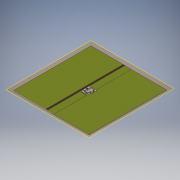
# Autodesk Inventor part: Umgebung
Saved by Autodesk Inventor 2019 (Build 230136000, 136)
## iProperties
Created: 2019-05-04
Part Number: Umgebung
Material: Generisch
Document SubType Name: Modeling
Designer: niede
Density: 1 g/cm^3
Appearance: Default
Author: niede
Autodesk Inventor part; units mm, degrees
ref_plane "YZ Plane" through (0, 0, 0) normal (1, 0, 0) x (0, 1, 0)
ref_plane "XZ Plane" through (0, 0, 0) normal (0, 1, 0) x (-1, 0, 0)
ref_plane "XY Plane" through (0, 0, 0) normal (0, 0, 1) x (1, 0, 0)
sketch "Skizze2" plane through (0, 0, 0) normal (0, 1, 0) x (-1, 0, 0)
  line L0 (0, 0) -> (11230, 0)
  line L1 (11230, 0) -> (11230, -6920)
  line L2 (11230, -6920) -> (10230, -6920)
  line L3 (10230, -6920) -> (10230, -17740)
  line L4 (10230, -17740) -> (11230, -17740)
  line L5 (11230, -17740) -> (11230, -17980)
  line L6 (11230, -17980) -> (2740, -17980)
  line L7 (2740, -17980) -> (2740, -14980)
  line L8 (2740, -14980) -> (-1250, -14980)
  line L9 (-1250, -14980) -> (-1250, -8870)
  line L10 (-1250, -8870) -> (1180, -8870)
  line L11 (1180, -8870) -> (1180, -4980)
  line L12 (1180, -4980) -> (0, -4980)
  line L13 (0, -4980) -> (0, 0)
  line L14 (111230, 100000) -> (-101250, 100000)
  line L15 (-101250, 100000) -> (-101250, -117980)
  line L16 (-101250, -117980) -> (111230, -117980)
  line L17 (111230, -117980) -> (111230, 100000)
  dimension "d0" = 11230
  dimension "d1" = 6920
  dimension "d2" = 1000
  dimension "d3" = 10820
  dimension "d4" = 240
  dimension "d5" = 8490
  dimension "d6" = 3000
  dimension "d7" = 3990
  dimension "d8" = 6110
  dimension "d9" = 2430
  dimension "d10" = 3890
  dimension "d11" = 1180
  dimension "d12" = 11230
  dimension "d13" = 6920
  dimension "d14" = 100000
  dimension "d15" = 100000
  dimension "d16" = 100000
  dimension "d17" = 100000
  constraints: 36 end point, 10 perpendicular, 2 horizontal, 2 parallel, 2 point on line, 2 vertical
  measures "d0" distance of L0.start L0.end
  measures "d1" distance of L0.end L1.end
  measures "d2" distance of L1.end L2.end
  measures "d3" distance of L2.end L3.end
  measures "d4" distance of L4.end L5.end
  measures "d5" distance of L5.end L6.end
  measures "d6" distance of L6.end L7.end
  measures "d7" distance of L7.end L8.end
  measures "d8" distance of L8.end L9.end
  measures "d9" distance of L9.end L10.end
  measures "d10" distance of L10.end L11.end
  measures "d11" distance of L11.end L12.end
  measures "d12" distance from line of point (0, 0) L1
  measures "d13" distance from line of point (0, 0) L2
  measures "d14" distance between parallel lines of L17 L1
  measures "d15" distance between parallel lines of L15 L9
  measures "d16" distance between parallel lines of L6 L16
  measures "d17" distance between parallel lines of L0 L14
extrude "Haus_Senkung" add sketch "Skizze2" along normal blind 1700
sketch "Skizze3" plane through (0, 1700, 0) normal (0, 1, 0) x (1, 0, 0)
  line L0 (1250, 8870) -> (-1180, 8870) projected
  line L1 (-1180, 8870) -> (-1180, 4980) projected
  line L2 (0, 4980) -> (-1180, 4980) projected
  line L3 (4500, 4980) -> (4500, 8870)
  line L4 (4500, 8870) -> (1250, 8870)
  line L5 (3000, 4980) -> (3000, 2880)
  line L6 (3000, 2880) -> (1800, 2880)
  line L7 (1800, 2880) -> (1800, 4980)
  line L8 (0, 4980) -> (1800, 4980)
  line L9 (3000, 4980) -> (4500, 4980)
  dimension "d20" = 4500
  dimension "d47" = 1500
  dimension "d48" = 1200
  dimension "d49" = 2100
  constraints: 14 end point, 8 perpendicular, 2 horizontal, 1 collinear
  measures "d20" distance of L2.start L3.start
  measures "d47" distance between parallel lines of L5 L3
  measures "d48" distance between parallel lines of L5 L7
  measures "d49" distance of L6.end L7.end
extrude "Terrasse_Senkung_1" cut sketch "Skizze3" against normal blind 1400
sketch "Skizze4" plane through (1250, 0, -14980) normal (-1, 0, 0) x (0, 0, 1)
  line L0 (6110, 300) -> (6110, 1700) projected
  line L1 (0, 1700) -> (6110, 1700) projected
  line L2 (0, 0) -> (0, 1700) projected
  line L3 (6110, 500) -> (5760, 500)
  line L4 (5760, 500) -> (5760, 700)
  line L5 (5760, 700) -> (5410, 700)
  line L6 (5410, 700) -> (5410, 900)
  line L7 (5410, 900) -> (5060, 900)
  line L8 (5060, 900) -> (5060, 1100)
  line L9 (5060, 1100) -> (4710, 1100)
  line L10 (4710, 1100) -> (4710, 1300)
  line L11 (4710, 1300) -> (700, 1300)
  line L12 (700, 1300) -> (700, 1500)
  line L13 (700, 1500) -> (350, 1500)
  line L14 (350, 1500) -> (350, 1700)
  point P0 (14980, 0)
  dimension "d23" = 200
  dimension "d24" = 200
  dimension "d25" = 350
  dimension "d29" = 350
  constraints: 24 end point, 10 perpendicular, 8 parallel, 2 point on line, 1 horizontal, 1 vertical
  measures "d23" distance of L5.end L6.end
  measures "d24" distance from line of L3 L0.start
  measures "d25" distance of L4.end L5.end
  measures "d29" distance between parallel lines of L2 L14
extrude "Terrasse_Treppe_Rechts" cut sketch "Skizze4" against normal blind 1200
sketch "Skizze8" plane through (0, 1700, 0) normal (0, 1, 0) x (1, 0, 0)
  line L0 (2450, 14630) -> (2450, 8870) projected
  line L1 (2450, 8870) -> (4500, 8870) projected
  line L2 (4500, 8870) -> (4500, 4980) projected
  line L3 (4500, 4980) -> (3000, 4980) projected
  line L4 (3000, 4980) -> (3000, 2880) projected
  line L5 (2450, 9870) -> (5500, 9870)
  line L6 (5500, 9870) -> (5500, 3980)
  line L7 (5500, 3980) -> (3300, 3980)
  line L8 (3300, 3980) -> (3300, 4980)
  dimension "d50" = 1000
  dimension "d51" = 1000
  dimension "d52" = 1000
  dimension "d53" = 300
  constraints: 8 end point, 3 perpendicular, 2 point on line, 1 horizontal
  measures "d50" distance between parallel lines of L1 L5
  measures "d51" distance between parallel lines of L2 L6
  measures "d52" distance between parallel lines of L3 L7
  measures "d53" distance between parallel lines of L4 L8
extrude "Terrasse_Senkung_2" cut sketch "Skizze8" against normal blind 700
sketch "Skizze5" plane through (-2740, 0, -14980) normal (0, 0, 1) x (1, 0, 0)
  line L0 (3990, 0) -> (0, 0) projected
  line L1 (0, 1700) -> (3990, 1700) projected
  line L2 (0, 0) -> (0, 1700) projected
  line L3 (1350, 500) -> (1350, 700)
  line L4 (1350, 700) -> (1700, 700)
  line L5 (1700, 700) -> (1700, 900)
  line L6 (1700, 900) -> (2050, 900)
  line L7 (2050, 900) -> (2050, 1100)
  line L8 (2050, 1100) -> (2400, 1100)
  line L9 (2400, 1100) -> (2400, 1300)
  line L10 (2400, 1300) -> (2750, 1300)
  line L11 (2750, 1300) -> (2750, 1500)
  line L12 (2750, 1500) -> (3100, 1500)
  line L13 (3100, 1500) -> (3100, 1700)
  line L14 (1350, 500) -> (1000, 500)
  line L15 (1000, 500) -> (1000, 300)
  line L16 (1000, 300) -> (0, 300)
  point P0 (2740, 0)
  dimension "d32" = 200
  dimension "d33" = 1000
  dimension "d34" = 300
  dimension "d35" = 350
  constraints: 28 end point, 12 perpendicular, 11 parallel, 2 point on line, 1 horizontal
  measures "d32" distance of L3.start L3.end
  measures "d33" distance of L15.end L16.end
  measures "d34" distance between parallel lines of L0 L16
  measures "d35" distance of L3.start L14.end
extrude "Plattform_Treppe" cut sketch "Skizze5" against normal blind 1000
sketch "Skizze9" plane through (3000, 1700, -4980) normal (-1, 0, 0) x (0, 0, 1)
  line L0 (0, 0) -> (2100, 0) projected
  line L1 (0, 0) -> (0, -1400) projected
  line L2 (0, -1400) -> (2100, -1400) projected
  line L3 (2100, 0) -> (2100, -1400) projected
  line L4 (0, -1200) -> (300, -1200)
  line L5 (300, -1200) -> (300, -1000)
  line L6 (300, -1000) -> (600, -1000)
  line L7 (600, -1000) -> (600, -800)
  line L8 (600, -800) -> (900, -800)
  line L9 (900, -800) -> (900, -600)
  line L10 (900, -600) -> (1200, -600)
  line L11 (1200, -600) -> (1200, -400)
  line L12 (1200, -400) -> (1500, -400)
  line L13 (1500, -400) -> (1500, -200)
  line L14 (1500, -200) -> (1800, -200)
  line L15 (1800, -200) -> (1800, 0)
  point P0 (4980, -1700)
  dimension "d56" = 200
  dimension "d57" = 300
  constraints: 24 end point, 11 perpendicular, 10 parallel, 2 point on line, 1 horizontal
  measures "d56" distance of L14.end L15.end
  measures "d57" distance of L4.start L4.end
extrude "Terrasse_Treppe_Links" add sketch "Skizze9" along normal blind 1200 contours L0 L3 L2 L1 L4 L5 L6 L7 L8 L9 L10 L11 L12 L13 L14 L15
sketch "Skizze14" plane through (0, 1700, 0) normal (0, 1, 0) x (1, 0, 0)
  line L0 (-2740, 17980) -> (-2740, 15980) projected
  line L1 (-2740, 15980) -> (360, 15980) projected
  line L2 (360, 15980) -> (360, 14980) projected
  line L3 (360, 14980) -> (1250, 14980) projected
  line L4 (1250, 14980) -> (1250, 14630) projected
  line L5 (1250, 14630) -> (2450, 14630) projected
  line L6 (2450, 14630) -> (2450, 9870) projected
  line L7 (-2740, 17980) -> (6260, 17980)
  line L8 (6260, 17980) -> (6260, 13580)
  line L9 (6260, 13580) -> (2450, 13580)
  line L10 (2450, 10270) -> (2450, 14280) projected
  point P0 (0, 0)
  dimension "d79" = 9000
  dimension "d80" = 4400
  constraints: 6 end point, 2 perpendicular, 1 horizontal, 1 point on line
  measures "d79" distance of L0.start L7.end
  measures "d80" distance of L7.end L8.end
extrude "Plattform_Erhebung" add sketch "Skizze14" along normal blind 200
sketch "Skizze10" plane through (0, 1700, 0) normal (0, 1, 0) x (1, 0, 0)
  line L0 (0, 4980) -> (0, 0) projected
  line L1 (0, 1500) -> (4000, 1500)
  line L2 (4000, 1500) -> (4000, -2500)
  line L3 (4000, -2500) -> (-300, -2500)
  line L4 (-300, -2500) -> (-300, 0)
  line L5 (-11230, 0) -> (0, 0) projected
  dimension "d60" = 4000
  dimension "d61" = 4000
  dimension "d62" = 4300
  dimension "d63" = 2500
  constraints: 8 end point, 3 perpendicular, 2 point on line, 1 horizontal
  measures "d60" distance of L1.start L1.end
  measures "d61" distance of L1.end L2.end
  measures "d62" distance of L2.end L3.end
  measures "d63" distance of L3.end L4.end
extrude "Holzterasse_Erhebung" add sketch "Skizze10" along normal blind 200
sketch "Skizze11" plane through (0, 1900, 0) normal (0, 1, 0) x (1, 0, 0)
  line L0 (0, 0) -> (-300, 0) projected
  line L1 (-300, 0) -> (-300, -2500) projected
  line L2 (0, 0) -> (0, -1800)
  line L3 (0, -1800) -> (-300, -1800)
  dimension "d66" = 1800
  constraints: 4 end point, 1 perpendicular, 1 point on line, 1 vertical
  measures "d66" distance of L0.start L2.end
extrude "Holzterasse_Wand" add sketch "Skizze11" along normal blind 2000
sketch "Skizze12" plane through (0, 1700, 0) normal (0, 1, 0) x (1, 0, 0)
  line L0 (-300, 0) -> (-11230, 0) projected
  line L1 (-11230, 0) -> (-11230, 6920) projected
  line L2 (-10230, 0) -> (-10230, -1400)
  line L3 (-10230, -1400) -> (-300, -1400)
  line L4 (-300, 0) -> (-300, -1800) projected
  point P0 (0, 0)
  dimension "d69" = 1400
  dimension "d70" = 1000
  constraints: 4 end point, 2 perpendicular, 2 point on line
  measures "d69" distance of L2.start L2.end
  measures "d70" distance between parallel lines of L1 L2
extrude "Steinbett_Absenkung" cut sketch "Skizze12" against normal blind 300
sketch "Skizze13" plane through (0, 0, -4980) normal (-1, 0, 0) x (0, 0, 1)
  line L0 (3480, 1700) -> (3130, 1700)
  line L1 (3130, 1700) -> (3130, 1900)
  line L2 (3130, 1900) -> (3480, 1900)
  line L3 (3480, 1900) -> (3480, 1700)
  line L4 (3130, 1900) -> (2780, 1900)
  line L5 (2780, 1900) -> (2780, 2100)
  line L6 (2780, 2100) -> (3130, 2100)
  line L7 (3130, 2100) -> (3130, 1900)
  line L8 (2780, 2100) -> (2430, 2100)
  line L9 (2430, 2100) -> (2430, 2300)
  line L10 (2430, 2300) -> (2780, 2300)
  line L11 (2780, 2300) -> (2780, 2100)
  line L12 (2430, 2300) -> (2080, 2300)
  line L13 (2080, 2300) -> (2080, 2500)
  line L14 (2080, 2500) -> (2430, 2500)
  line L15 (2430, 2500) -> (2430, 2300)
  line L16 (2080, 2500) -> (1730, 2500)
  line L17 (1730, 2500) -> (1730, 2700)
  line L18 (1730, 2700) -> (2080, 2700)
  line L19 (2080, 2700) -> (2080, 2500)
  line L20 (1730, 2700) -> (1380, 2700)
  line L21 (1380, 2700) -> (1380, 2900)
  line L22 (1380, 2900) -> (1730, 2900)
  line L23 (1730, 2900) -> (1730, 2700)
  line L24 (1380, 2900) -> (0, 2900)
  line L25 (0, 2900) -> (0, 3100)
  line L26 (0, 3100) -> (1380, 3100)
  line L27 (1380, 3100) -> (1380, 2900)
  dimension "d73" = 200
  dimension "d74" = 350
  dimension "d75" = 1380
  constraints: 56 end point, 14 parallel, 11 equal length, 7 horizontal, 7 perpendicular
  measures "d73" distance of L0.end L1.end
  measures "d74" distance of L21.end L22.end
  measures "d75" distance of L25.end L26.end
extrude "Treppe_Erdgeschoss" add sketch "Skizze13" against normal blind 1200
sketch "Skizze15" plane through (0, 1700, 0) normal (0, 1, 0) x (1, 0, 0)
  line L0 (-10230, -1400) -> (-10230, 0) projected
  line L1 (-10230, 0) -> (-11230, 0) projected
  line L2 (-11230, 0) -> (-11230, 6920) projected
  line L3 (-11230, 6920) -> (-10230, 6920) projected
  line L4 (-10230, 6920) -> (-10230, 17740) projected
  line L5 (-10230, 17740) -> (-11230, 17740) projected
  line L6 (-111230, -100000) -> (101250, -100000) projected
  line L7 (101250, 117980) -> (-111230, 117980) projected
  line L8 (-111230, 117980) -> (-111230, -100000) projected
  line L9 (-10230, -4900) -> (-5730, -4900)
  line L10 (-5730, -4900) -> (-5730, -8350)
  line L11 (-5730, -8350) -> (-15480, -8350)
  line L12 (-10230, -1700) -> (-10230, -4900)
  line L13 (-11230, 17980) -> (-11230, 17740) projected
  line L14 (-15480, 17980) -> (-11230, 17980)
  line L15 (-15480, -100000) -> (-15480, -8350)
  line L16 (-15480, 17980) -> (-15480, 117980)
  line L17 (-300, -1400) -> (-10230, -1400) projected
  line L18 (-10230, -1700) -> (-9230, -1700)
  line L19 (-9230, -1700) -> (-9230, -1400)
  point P0 (0, 0)
  dimension "d84" = 3450
  dimension "d85" = 3500
  dimension "d86" = 4500
  dimension "d87" = 4250
  dimension "d132" = 1000
  dimension "d133" = 300
  constraints: 18 end point, 9 perpendicular, 3 point on line, 2 collinear, 2 horizontal
  measures "d84" distance of L9.end L10.end
  measures "d85" distance of L9.start L0.start
  measures "d86" distance between parallel lines of L10 L12
  measures "d87" distance between parallel lines of L15 L2
  measures "d132" distance of L12.start L18.end
  measures "d133" distance of L18.end L19.end
extrude "Straße_Erhöhung" add sketch "Skizze15" along normal blind 900
ref_plane "Ebene_Rasensteigung" through (2450, 1700, -10227.1121) normal (-0.0501321, -0.9987426, 0) x (0, 0, 1)
sketch "Skizze18" plane through (2450, 1700, -10227.1121) normal (-0.0501321, -0.9987426, 0) x (0, 0, 1)
  line L0 (-7752.8879, -3795.1829) -> (-7752.8879, 5193.5005) projected
  line L1 (-7752.8879, 17952.5736) -> (-107752.8879, 17952.5736) projected
  line L2 (-7752.8879, 14.6347) -> (-107752.8879, 14.6347)
  line L3 (-107752.8879, 14.6347) -> (-107752.8879, 17952.5736)
  line L4 (-107752.8879, 17952.5736) -> (-7752.8879, 17952.5736)
  line L5 (-7752.8879, 17952.5736) -> (-7752.8879, 14.6347)
  line L6 (18577.1121, 8169.7144) -> (18577.1121, 17907.4548) projected
  line L7 (110227.1121, 113451.8338) -> (110227.1121, -98760.9931) projected
  line L8 (18577.1121, 17907.4548) -> (110227.1121, 17907.4548)
  line L9 (110227.1121, 17907.4548) -> (110227.1121, 14.6347)
  line L10 (110227.1121, 14.6347) -> (18577.1121, 14.6347)
  line L11 (18577.1121, 14.6347) -> (18577.1121, 17907.4548)
  point P0 (10227.1121, 2361.6948)
  dimension "d91" = 17937.9389
  constraints: 16 end point, 4 parallel, 3 point on line, 2 horizontal, 2 perpendicular
  measures "d91" distance between parallel lines of L1 L10
extrude "Rasen_Erhebung" add sketch "Skizze18" along normal blind 1200
sketch "Skizze19" plane through (0, 2600, 0) normal (0, 1, 0) x (1, 0, 0)
  line L0 (-10230, -4900) -> (-10230, 0) projected
  line L1 (-10230, 0) -> (-11230, 0) projected
  line L2 (-11230, 0) -> (-11230, 6920) projected
  line L3 (-11230, 6920) -> (-10230, 6920) projected
  line L4 (-10230, 6920) -> (-10230, 17740) projected
  line L5 (-10230, 17740) -> (-11230, 17740) projected
  line L6 (-11230, 17740) -> (-11230, 17980) projected
  line L7 (-11230, 17980) -> (-15480, 17980) projected
  line L8 (-15480, -8350) -> (-5730, -8350) projected
  line L9 (-5730, -8350) -> (-5730, -4900) projected
  line L10 (-5730, -4900) -> (-10230, -4900) projected
  line L11 (-15480, 17980) -> (-15480, -8350)
  point P0 (0, 0)
  constraints: 2 end point, 1 vertical
extrude "Haus_Nord_Erhebung" add sketch "Skizze19" along normal blind 100
sketch "Skizze20" plane through (0, 2700, 0) normal (0, 1, 0) x (1, 0, 0)
  line L0 (-10230, 0) -> (-11230, 0) projected
  line L1 (-11230, 0) -> (-11230, 6920) projected
  line L2 (-11230, 6920) -> (-10230, 6920) projected
  line L3 (-10230, 6920) -> (-10230, 17740) projected
  line L4 (-15480, 17980) -> (-15480, -8350) projected
  line L5 (-11230, 400) -> (-12430, 400)
  line L6 (-12430, 400) -> (-12430, -400)
  line L7 (-12430, -400) -> (-15480, -400)
  line L8 (-15480, -400) -> (-15480, 8420)
  line L9 (-14230, 8420) -> (-14230, 6920)
  line L10 (-14230, 6920) -> (-12230, 6920)
  line L11 (-12230, 6920) -> (-12230, 8420)
  line L12 (-15480, 8420) -> (-14230, 8420)
  line L13 (-12230, 8420) -> (-10230, 8420)
  point P0 (0, 0)
  dimension "d97" = 1200
  dimension "d99" = 800
  dimension "d100" = 400
  dimension "d101" = 1500
  dimension "d102" = 2000
  dimension "d103" = 2000
  constraints: 18 end point, 10 perpendicular, 4 point on line, 2 collinear
  measures "d97" distance of L5.start L5.end
  measures "d99" distance of L5.end L6.end
  measures "d100" distance between parallel lines of L7 L0
  measures "d101" distance of L9.start L9.end
  measures "d102" distance of L9.end L10.end
  measures "d103" distance of L11.end L13.end
extrude "Haus_Nord_Rasen_Erhebung" add sketch "Skizze20" along normal blind 200
sketch "Skizze21" plane through (0, 2700, 0) normal (0, 1, 0) x (1, 0, 0)
  line L0 (-14230, 8420) -> (-14230, 6920) projected
  line L1 (-14230, 6920) -> (-12230, 6920) projected
  line L2 (-12230, 6920) -> (-12230, 8420) projected
  line L3 (-12230, 8420) -> (-13230, 8420)
  line L4 (-13230, 8420) -> (-13230, 8720)
  line L5 (-13230, 8720) -> (-14230, 8720)
  line L6 (-14230, 8720) -> (-14230, 8420)
  point P0 (0, 0)
  dimension "d106" = 1000
  dimension "d107" = 300
  constraints: 8 end point, 3 perpendicular, 1 horizontal
  measures "d106" distance of L2.end L3.end
  measures "d107" distance of L3.end L4.end
extrude "Haus_Nord_Beet_Erhebung" add sketch "Skizze21" along normal blind 600
sketch "Skizze23" plane through (0, 2900, 0) normal (0, 1, 0) x (1, 0, 0)
  line L0 (-11230, 6920) -> (-10230, 6920) projected
  line L1 (-10230, 6920) -> (-10230, 8420) projected
  line L2 (-10230, 8420) -> (-12230, 8420) projected
  line L3 (-12230, 8420) -> (-12230, 6920) projected
  line L4 (-10230, 6920) -> (-11230, 6920) projected
  line L5 (-12230, 6920) -> (-11230, 6920)
  point P0 (0, 0)
  constraints: 2 end point, 1 horizontal
extrude "Haus_Nord_Stufe_Erhebung" add sketch "Skizze23" along normal blind 200
sketch "Skizze24" plane through (0, 3100, 0) normal (0, 1, 0) x (1, 0, 0)
  line L0 (-10230, 8420) -> (-10230, 17740) projected
  line L1 (-10230, 8420) -> (-11230, 8420)
  line L2 (-11230, 8420) -> (-11230, 7920)
  line L3 (-11230, 7920) -> (-10230, 7920)
  line L4 (-10230, 7920) -> (-10230, 8420)
  point P0 (0, 0)
  dimension "d112" = 1000
  dimension "d113" = 500
  constraints: 8 end point, 2 parallel, 1 horizontal, 1 perpendicular
  measures "d112" distance of L3.end L2.end
  measures "d113" distance of L1.end L2.end
extrude "Haus_Nord_Stufe_Sims_Erhebung" add sketch "Skizze24" along normal blind 1000
sketch "Skizze25" plane through (0, 3300, 0) normal (0, 1, 0) x (1, 0, 0)
  line L0 (-14230, 8720) -> (-14230, 6920) projected
  line L1 (-12230, 6920) -> (-12230, 8420) projected
  line L2 (-12230, 8420) -> (-13230, 8420) projected
  line L3 (-13230, 8420) -> (-13230, 8720) projected
  line L4 (-13230, 8720) -> (-14230, 8720) projected
  line L5 (-14230, 8120) -> (-12230, 8120)
  line L6 (-12230, 6920) -> (-12230, 8420) projected
  point P0 (0, 0)
  dimension "d116" = 300
  constraints: 2 end point, 2 point on line, 1 perpendicular
  measures "d116" distance between parallel lines of L5 L2
extrude "Haus_Nord_Müll_Erhebung_1" add sketch "Skizze25" along normal blind 400
sketch "Skizze26" plane through (0, 3700, 0) normal (0, 1, 0) x (1, 0, 0)
  line L0 (-14230, 8720) -> (-14230, 8120) projected
  line L1 (-14230, 8120) -> (-12230, 8120) projected
  line L2 (-13230, 8420) -> (-13230, 8720) projected
  line L3 (-13230, 8720) -> (-14230, 8720) projected
  line L4 (-13230, 8420) -> (-13230, 8120)
  point P0 (0, 0)
  constraints: 2 end point, 1 midpoint
extrude "Haus_Nord_Müll_Erhebung_2" add sketch "Skizze26" along normal blind 400
sketch "Skizze27" plane through (0, 3300, 0) normal (0, 1, 0) x (1, 0, 0)
  line L0 (-12230, 8120) -> (-14230, 8120) projected
  line L1 (-14230, 8120) -> (-14230, 6920) projected
  line L2 (-14230, 6920) -> (-12230, 6920) projected
  line L3 (-12230, 6920) -> (-12230, 8120) projected
  line L4 (-12530, 8120) -> (-13930, 8120)
  line L5 (-13930, 8120) -> (-13930, 7220)
  line L6 (-13930, 7220) -> (-12530, 7220)
  line L7 (-12530, 7220) -> (-12530, 8120)
  point P0 (0, 0)
  dimension "d121" = 300
  dimension "d122" = 300
  dimension "d123" = 300
  constraints: 8 end point, 2 parallel, 1 horizontal, 1 perpendicular, 1 point on line
  measures "d121" distance between parallel lines of L3 L7
  measures "d122" distance between parallel lines of L2 L6
  measures "d123" distance between parallel lines of L1 L5
extrude "Haus_Nord_Beet_Rand_Erhebung" add sketch "Skizze27" along normal blind 100 contours L3 L2 L1 L0 L5 L6 L7
sketch "Skizze28" plane through (0, 2700, 0) normal (0, 1, 0) x (1, 0, 0)
  line L0 (-13230, 8420) -> (-10230, 8420) projected
  line L1 (-10230, 8420) -> (-10230, 17740) projected
  line L2 (-10230, 17740) -> (-11230, 17740) projected
  line L3 (-11230, 17740) -> (-11230, 17980) projected
  line L4 (-11230, 17980) -> (-15480, 17980) projected
  line L5 (-15480, 17980) -> (-15480, 8420) projected
  line L6 (-15480, 8420) -> (-14230, 8420) projected
  line L7 (-14230, 8420) -> (-14230, 8720) projected
  line L8 (-14230, 8720) -> (-13230, 8720) projected
  line L9 (-13230, 8720) -> (-13230, 8420) projected
  point P0 (0, 0)
extrude "Haus_Einfahr_Erhebung" add sketch "Skizze28" along normal blind 400
sketch "Skizze29" plane through (-11230, 3100, -17980) normal (0, 0, -1) x (-1, 0, 0)
  line L0 (-1000, 0) -> (0, 0) projected
  line L1 (-1000, -3100) -> (-1000, 0) projected
  line L2 (-1000, 0) -> (4250, 0)
  line L3 (4250, -500) -> (4250, 0) projected
  line L4 (4250, -400) -> (4250, -200) projected
  line L5 (4250, 0) -> (4250, -400)
  line L6 (1000, 0) -> (-1000, 0) projected
  line L7 (4250, -400) -> (-1000, 0)
  point P0 (-11230, -3100)
  constraints: 6 end point, 1 collinear, 1 horizontal
extrude "Haus_Einfahr_Verbesserung_1" cut sketch "Skizze29" against normal blind 9260
sketch "Skizze30" plane through (-14230, 3100, -8720) normal (0, 0, -1) x (-1, 0, 0)
  line L0 (-4000, 0) -> (-1000, 0) projected
  line L1 (1250, -400) -> (-4000, 0) projected
  line L2 (1250, 0) -> (1250, -400) projected
  line L3 (0, 0) -> (1250, 0) projected
  line L4 (-1000, 0) -> (-1000, -228.5714)
  line L5 (0, 0) -> (0, -304.7619)
  point P0 (-14230, -3100)
  constraints: 4 end point, 2 point on line, 1 parallel, 1 vertical
extrude "Haus_Einfahr_Verbesserung_2" cut sketch "Skizze30" against normal blind 300
sketch "Skizze32" plane through (0, 2700, 0) normal (0, 1, 0) x (1, 0, 0)
  line L0 (-12430, -400) -> (-15480, -400) projected
  line L1 (-15480, -400) -> (-15480, -8350) projected
  line L2 (-15480, -8350) -> (-5730, -8350) projected
  line L3 (-5730, -8350) -> (-5730, -4900) projected
  line L4 (-5730, -4900) -> (-10230, -4900) projected
  line L5 (-10230, -4900) -> (-10230, 0) projected
  line L6 (-10230, 0) -> (-11230, 0) projected
  line L7 (-11230, 0) -> (-11230, 400) projected
  line L8 (-11230, 400) -> (-12430, 400) projected
  line L9 (-12430, 400) -> (-12430, -400) projected
  point P0 (0, 0)
extrude "Haus_Carport_Verbesserung" cut sketch "Skizze32" against normal blind 100
sketch "Skizze33" plane through (-10230, 1700, 1700) normal (0, 0, 1) x (1, 0, 0)
  line L0 (1000, 0) -> (0, 0) projected
  line L1 (0, 900) -> (0, -300) projected
  line L2 (0, 900) -> (1000, 0)
  point P0 (10230, -1700)
  constraints: 2 end point
extrude "Haus_Carport_Steigung" add sketch "Skizze33" along normal blind 1200
sketch "Skizze34" plane through (0, 2600, 0) normal (0, 1, 0) x (1, 0, 0)
  line L0 (-15480, -400) -> (-15480, 17980) projected
  line L1 (-15480, 17980) -> (-15480, 117980) projected
  line L2 (-15480, 117980) -> (-111230, 117980) projected
  line L3 (-111230, -100000) -> (-15480, -100000) projected
  line L4 (-15480, -100000) -> (-15480, -8350) projected
  line L5 (-15480, -400) -> (-12430, -400) projected
  line L6 (-15480, -400) -> (-15480, -8350)
  line L7 (-20480, 117980) -> (-20480, -100000)
  point P0 (0, 0)
  dimension "d138" = 5000
  constraints: 4 end point, 2 point on line, 1 perpendicular, 1 vertical
  measures "d138" distance between parallel lines of L4 L7
extrude "Straße_Senkung" cut sketch "Skizze34" against normal blind 100
sketch "Sketch36" plane through (0, 1700, 0) normal (0, 1, 0) x (1, 0, 0)
  line L0 (-5730, -8350) -> (-2280, -8350)
  line L1 (-2280, -8350) -> (-2280, -4900)
  line L2 (-2280, -4900) -> (-5730, -4900)
  line L3 (-5730, -4900) -> (-5730, -8350)
  line L4 (-2480, -8150) -> (-5530, -8150)
  line L5 (-5530, -8150) -> (-5530, -5100)
  line L6 (-5530, -5100) -> (-2480, -5100)
  line L7 (-2480, -5100) -> (-2480, -8150)
  point P0 (0, 0)
  dimension "d146" = 3450
  dimension "d147" = 3450
  dimension "d148" = 200
  dimension "d149" = 3050
  dimension "d150" = 200
  constraints: 16 end point, 4 parallel, 3 perpendicular, 2 horizontal
  measures "d146" distance of L2.end L1.end
  measures "d147" distance of L0.end L1.end
  measures "d148" distance between parallel lines of L7 L1
  measures "d149" distance of L4.start L4.end
  measures "d150" distance between parallel lines of L0 L4
extrude "Carport_Erhebung" add sketch "Sketch36" along normal blind 900
sketch "Sketch37" plane through (0, 2600, 0) normal (0, 1, 0) x (1, 0, 0)
  line L0 (-2480, -5100) -> (-2480, -8150) projected
  line L1 (-5530, -5100) -> (-2480, -5100) projected
  line L2 (-2480, -8150) -> (-5530, -8150)
  line L3 (-5530, -8150) -> (-5530, -5100)
  line L4 (-5530, -5100) -> (-2480, -5100)
  line L5 (-2480, -5100) -> (-2480, -8150)
  line L6 (-2280, -4900) -> (-2280, -8350) projected
  line L7 (-10230, -4900) -> (-2280, -4900) projected
  line L8 (-2280, -8350) -> (-5730, -8350)
  line L9 (-5730, -8350) -> (-5730, -4900)
  line L10 (-5730, -4900) -> (-2280, -4900)
  line L11 (-2280, -4900) -> (-2280, -8350)
  line L12 (-2280, -8350) -> (-15434.9379, -8350) projected
  line L13 (-8230, -8350) -> (-8430, -8350)
  line L14 (-8430, -8350) -> (-8430, -8150)
  line L15 (-8430, -8150) -> (-8230, -8150)
  line L16 (-8230, -8150) -> (-8230, -8350)
  line L17 (-8230, -4900) -> (-8430, -4900)
  line L18 (-8430, -4900) -> (-8430, -5100)
  line L19 (-8430, -5100) -> (-8230, -5100)
  line L20 (-8230, -5100) -> (-8230, -4900)
  line L21 (-10930, -4900) -> (-11130, -4900)
  line L22 (-11130, -4900) -> (-11130, -5500)
  line L23 (-11130, -5500) -> (-10930, -5500)
  line L24 (-10930, -5500) -> (-10930, -4900)
  line L25 (-10930, -8350) -> (-11130, -8350)
  line L26 (-11130, -8350) -> (-11130, -8150)
  line L27 (-11130, -8150) -> (-10930, -8150)
  line L28 (-10930, -8150) -> (-10930, -8350)
  point P0 (0, 0)
  dimension "d153" = 3450
  dimension "d154" = 200
  dimension "d155" = 200
  dimension "d156" = 600
  dimension "d157" = 2500
  dimension "d158" = 2500
  constraints: 48 end point, 12 parallel, 12 point on line, 6 horizontal, 6 perpendicular
  measures "d153" distance of L9.end L10.end
  measures "d154" distance of L14.end L15.end
  measures "d155" distance of L23.end L22.end
  measures "d156" distance of L21.end L22.end
  measures "d157" distance between parallel lines of L9 L16
  measures "d158" distance between parallel lines of L28 L14
extrude "Carport_Erhebung_2" add sketch "Sketch37" along normal blind 2000
ref_plane "Ebene_Carport_Dach" through (-2280, 4600, 8350) normal (0, 1, 0) x (0, 0, -1)
sketch "Sketch38" plane through (-2280, 4600, 8350) normal (0, 1, 0) x (0, 0, -1)
  line L0 (3450, 0) -> (0, 0) projected
  line L1 (0, 0) -> (3750, 0)
  line L2 (3750, 0) -> (3750, 9150)
  line L3 (3750, 9150) -> (0, 9150)
  line L4 (0, 9150) -> (0, 0)
  line L5 (200, 8850) -> (0, 8850) projected
  line L6 (3450, 8650) -> (3450, 8850) projected
  point P0 (8350, -2280)
  dimension "d161" = 300
  dimension "d162" = 300
  constraints: 8 end point, 2 parallel, 1 horizontal, 1 perpendicular
  measures "d161" distance between parallel lines of L3 L5
  measures "d162" distance between parallel lines of L2 L6
extrude "Carport_Dach_Erhebung" add sketch "Sketch38" along normal blind 200
sketch "Sketch39" plane through (-10230, 1700, 4900) normal (0, 0, -1) x (-1, 0, 0)
  line L0 (0, 0) -> (-7950, 0) projected
  line L1 (-6500, 0) -> (-5500, 0)
  line L2 (-5500, 0) -> (-5500, 2000)
  line L3 (-5500, 2000) -> (-6500, 2000)
  line L4 (-6500, 2000) -> (-6500, 0)
  line L5 (-4500, 900) -> (-4500, 2900) projected
  point P0 (-10230, -1700)
  dimension "d165" = 1000
  dimension "d166" = 1000
  dimension "d167" = 2000
  constraints: 8 end point, 2 parallel, 1 horizontal, 1 perpendicular, 1 point on line
  measures "d165" distance between parallel lines of L5 L2
  measures "d166" distance between parallel lines of L2 L4
  measures "d167" distance of L3.end L1.start
extrude "Carport_Tür_Senkung" cut sketch "Sketch39" against normal blind 200
